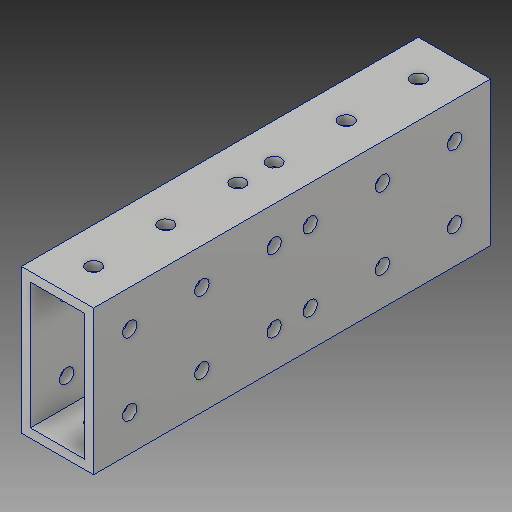
# Autodesk Inventor part: 5.5 2x2
Saved by Autodesk Inventor 2018 (Build 220112000, 112)
## iProperties
Created: 2018-09-23
Part Number: 5.5 2x2
Material: Aluminum 6061
Document SubType Name: Modeling
Designer: maste
Density: 2.7 g/cm^3
Appearance: Aluminum - Flat
Author: maste
Autodesk Inventor part; units mm, degrees
ref_plane "YZ Plane" through (0, 0, 0) normal (1, 0, 0) x (0, 1, 0)
ref_plane "XZ Plane" through (0, 0, 0) normal (0, 1, 0) x (-1, 0, 0)
ref_plane "XY Plane" through (0, 0, 0) normal (0, 0, 1) x (1, 0, 0)
sketch "Sketch1" plane through (0, 0, 0) normal (0, 0, 1) x (1, 0, 0)
  line L0 (0, 0) -> (25.4, 0)
  line L1 (25.4, 0) -> (25.4, 50.8)
  line L2 (25.4, 50.8) -> (0, 50.8)
  line L3 (0, 50.8) -> (0, 0)
  line L4 (3.175, 3.175) -> (22.225, 3.175)
  line L5 (22.225, 3.175) -> (22.225, 47.625)
  line L6 (22.225, 47.625) -> (3.175, 47.625)
  line L7 (3.175, 47.625) -> (3.175, 3.175)
  dimension "d0" = 25.4
  dimension "d1" = 50.8
  dimension "d2" = 3.175
  dimension "d3" = 3.175
  dimension "d4" = 3.175
  dimension "d5" = 3.175
  constraints: 16 end point, 4 parallel, 2 horizontal, 2 perpendicular
  measures "d0" distance of L2.end L1.end
  measures "d1" distance of L1.end L0.end
  measures "d2" distance between parallel lines of L2 L6
  measures "d3" distance between parallel lines of L0 L4
  measures "d4" distance between parallel lines of L1 L5
  measures "d5" distance between parallel lines of L3 L7
extrude "Extrusion1" add sketch "Sketch1" along normal blind 139.7
sketch "Sketch2" plane through (25.4, 0, 0) normal (1, 0, 0) x (0, 0, -1)
  line L0 (0, 0) -> (0, 50.8) projected
  line L1 (0, 0) -> (0, 12.7)
  line L2 (0, 12.7) -> (-139.7, 12.7)
  line L3 (-139.7, 47.625) -> (-139.7, 3.175) projected
  line L4 (-139.7, 0) -> (-139.7, 50.8) projected
  line L5 (-139.7, 50.8) -> (-139.7, 38.1)
  line L6 (-139.7, 38.1) -> (0, 38.1)
  line L7 (-139.7, 38.1) -> (-127, 38.1)
  line L8 (-127, 38.1) -> (-127, 12.7)
  line L9 (0, 38.1) -> (-12.7, 38.1)
  line L10 (-12.7, 38.1) -> (-12.7, 12.7)
  line L11 (-12.7, 38.1) -> (-38.1, 38.1)
  line L12 (-38.1, 38.1) -> (-63.5, 38.1)
  line L13 (-127, 38.1) -> (-101.6, 38.1)
  line L14 (-101.6, 38.1) -> (-76.2, 38.1)
  circle A0 centre (-127, 38.1) radius 2.54
  circle A1 centre (-127, 12.7) radius 2.54
  circle A2 centre (-101.6, 38.1) radius 2.54
  circle A3 centre (-76.2, 38.1) radius 2.54
  circle A4 centre (-63.5, 38.1) radius 2.54
  circle A5 centre (-38.1, 38.1) radius 2.54
  circle A6 centre (-12.7, 38.1) radius 2.54
  circle A7 centre (-12.7, 12.7) radius 2.54
  circle A8 centre (-38.1, 12.7) radius 2.54
  circle A9 centre (-63.5, 12.7) radius 2.54
  circle A10 centre (-76.2, 12.7) radius 2.54
  circle A11 centre (-101.6, 12.7) radius 2.54
  dimension "d8" = 12.7
  dimension "d9" = 12.7
  dimension "d10" = 12.7
  dimension "d11" = 12.7
  dimension "d12" = 25.4
  dimension "d13" = 25.4
  dimension "d14" = 25.4
  dimension "d15" = 25.4
  dimension "d16" = 5.08
  constraints: 24 end point, 16 point on line, 12 centre point, 8 coincident, 4 perpendicular
  measures "d8" distance of L0.start L1.end
  measures "d9" distance of L4.end L5.end
  measures "d10" distance of L5.end L7.end
  measures "d11" distance of L6.end L9.end
  measures "d12" distance of L9.end L11.end
  measures "d13" distance of L11.end L12.end
  measures "d14" distance of L7.end L13.end
  measures "d15" distance of L13.end L14.end
  measures "d16" diameter of A0
extrude "Extrusion2" cut sketch "Sketch2" against normal blind 25.4 contours A7 L2 | L2 L10 A7 | A6 L10 L6 | L6 A6 | L2 A7 L10 | L10 A6 L6 | A8 L2 | L2 A8 | A5 L6 | L6 A5 | A9 L2 | L2 A9 | A4 L6 | L6 A4 | A10 L2 | L2 A10 | A3 L6 | L6 A3 | A11 L2 | L2 A11 | A2 L6 | L6 A2 | A1 L2 | L2 L8 A1 | A0 L8 L6 | L6 A0 | L2 A1 L8 | L8 A0 L6
sketch "Sketch3" plane through (0, 50.8, 0) normal (0, 1, 0) x (1, 0, 0)
  line L0 (3.175, 0) -> (22.225, 0) projected
  line L1 (12.7, 0) -> (12.7, -139.7)
  line L2 (12.7, -139.7) -> (12.7, -127)
  line L3 (12.7, -127) -> (12.7, -101.6)
  line L4 (12.7, -101.6) -> (12.7, -76.2)
  line L5 (12.7, 0) -> (12.7, -12.7)
  line L6 (12.7, -12.7) -> (12.7, -38.1)
  line L7 (12.7, -38.1) -> (12.7, -63.5)
  circle A0 centre (12.7, -12.7) radius 2.54
  circle A1 centre (12.7, -38.1) radius 2.54
  circle A2 centre (12.7, -63.5) radius 2.54
  circle A3 centre (12.7, -76.2) radius 2.54
  circle A4 centre (12.7, -101.6) radius 2.54
  circle A5 centre (12.7, -127) radius 2.54
  point P0 (0, 0)
  dimension "d19" = 12.7
  dimension "d20" = 25.4
  dimension "d21" = 25.4
  dimension "d22" = 12.7
  dimension "d23" = 25.4
  dimension "d24" = 25.4
  dimension "d25" = 5.08
  constraints: 14 end point, 6 centre point, 6 coincident, 6 point on line, 1 midpoint, 1 vertical
  measures "d19" distance of L1.end L2.end
  measures "d20" distance of L2.end L3.end
  measures "d21" distance of L3.end L4.end
  measures "d22" distance of L1.start L5.end
  measures "d23" distance of L5.end L6.end
  measures "d24" distance of L6.end L7.end
  measures "d25" diameter of A0
extrude "Extrusion3" cut sketch "Sketch3" against normal blind 111.125
body "Solid1"
